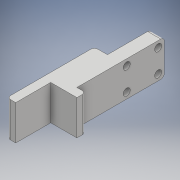
# Autodesk Inventor part: Esteira - Carro
Saved by Autodesk Inventor 2017 (Build 210142000, 142)
## iProperties
Created: 2020-09-19
Part Number: Esteira - Carro
Material: Generic
Document SubType Name: Modeling
Designer: ale
Density: 1 g/cm^3
Appearance: Default
Author: ale
Autodesk Inventor part; units mm, degrees
ref_plane "YZ Plane" through (0, 0, 0) normal (1, 0, 0) x (0, 1, 0)
ref_plane "XZ Plane" through (0, 0, 0) normal (0, 1, 0) x (-1, 0, 0)
ref_plane "XY Plane" through (0, 0, 0) normal (0, 0, 1) x (1, 0, 0)
sketch "Sketch1" plane through (0, 0, 0) normal (0, 0, 1) x (1, 0, 0)
  line L0 (0, -20) -> (0, 0)
  line L1 (0, 0) -> (15, 0)
  line L2 (-5, -20) -> (-5, 5)
  line L3 (-5, 5) -> (15, 5)
  line L4 (0, -20) -> (-5, -20)
  line L5 (15, 5) -> (15, 0)
  dimension "d0" = 15
  dimension "d1" = 20
  dimension "d2" = 5
  constraints: 12 end point, 3 perpendicular, 1 horizontal, 1 vertical, 1 other
  measures "d0" distance of L0.end L1.end
  measures "d1" distance of L0.start L0.end
  measures "d2" distance between parallel lines of L0 L2
extrude "Extrusion1" add sketch "Sketch1" along normal blind 20
sketch "Sketch2" plane through (-5, 5, 0) normal (0, 1, 0) x (1, 0, 0)
  line L0 (0, 0) -> (20, 0) projected
  line L1 (20, -20) -> (0, -20) projected
  line L2 (0, 0) -> (0, -20)
  line L3 (15, 0) -> (15, -20)
  line L4 (0, 0) -> (15, 0)
  line L5 (20, 0) -> (5, 0) projected
  line L6 (15, -20) -> (0, -20)
  line L7 (0, 0) -> (0, -20) projected
  dimension "d7" = 0
  dimension "d8" = 15
  constraints: 8 end point, 2 collinear
  measures "d7" distance between parallel lines of L7 L2
  measures "d8" distance between parallel lines of L7 L3
extrude "Extrusion2" add sketch "Sketch2" along normal blind 25
sketch "Sketch3" plane through (-5, 30, 0) normal (0, 1, 0) x (1, 0, 0)
  line L0 (15, 0) -> (15, -20) projected
  line L1 (15, 0) -> (7.5, 0)
  line L2 (7.5, 0) -> (7.5, -20)
  line L3 (7.5, -20) -> (15, -20)
  line L4 (15, -20) -> (15, 0)
  point P0 (5, 0)
  dimension "d11" = 7.5
  dimension "d12" = 20
  constraints: 8 end point, 2 parallel, 1 horizontal, 1 perpendicular
  measures "d11" distance of L3.end L2.end
  measures "d12" distance of L2.end L1.end
extrude "Extrusion3" add sketch "Sketch3" along normal blind 25
sketch "Sketch4" plane through (2.5, 30, 0) normal (-1, 0, 0) x (0, 0, 1)
  line L0 (0, 25) -> (20, 25) projected
  line L1 (10, 25) -> (10, 0)
  line L2 (20, 0) -> (0, 0) projected
  line L3 (0, 0) -> (0, 25) projected
  line L4 (0, 12.5) -> (20, 12.5)
  line L5 (20, -25) -> (20, 25) projected
  circle A0 centre (3.5, 21.5) radius 2
  circle A1 centre (16.5, 21.5) radius 2
  circle A2 centre (3.5, 3.5) radius 2
  circle A3 centre (16.5, 3.5) radius 2
  point P0 (0, -30)
  dimension "d15" = 4
  dimension "d16" = 3.5
  dimension "d17" = 3.5
  constraints: 4 centre point, 4 end point, 3 midpoint, 3 symmetric about line, 1 horizontal, 1 point on line, 3 other
  measures "d15" diameter of A0
  measures "d16" distance from line of L3 A0.centre
  measures "d17" distance from line of L0 A0.centre
hole "Hole1" at (2.5, 51.5, 3.5) at (2.5, 51.5, 16.5) at (2.5, 33.5, 16.5) at (2.5, 33.5, 3.5) direction (1, 0, 0) diameter 4 end through all
fillet "Fillet1" radius 2 5 edges at (-5, 30, 10) (6.25, 55, 0) (6.25, 55, 20) (15, 5, 10) (-5, -20, 10)
body "Solid1"
